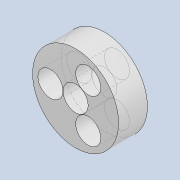
# Autodesk Inventor part: 原動節-ヘッケン接続部v2
Saved by Autodesk Inventor 2020 (Build 240168000, 168)
## iProperties
Created: 2020-06-16
Part Number: 原動節-ヘッケン接続部v2
Material: アルミニウム 2014-T4
Document SubType Name: Modeling
Designer: happy
Density: 2.8 g/cm^3
Appearance: サテン
Mass: 0.939484 g
Surface Area: 4.6873 cm^2
Volume: 0.33553 cm^3
Author: happy
Autodesk Inventor part; units mm, degrees
ref_plane "YZ Plane" through (0, 0, 0) normal (1, 0, 0) x (0, 1, 0)
ref_plane "XZ Plane" through (0, 0, 0) normal (0, 1, 0) x (-1, 0, 0)
ref_plane "XY Plane" through (0, 0, 0) normal (0, 0, 1) x (1, 0, 0)
sketch "スケッチ1" plane through (0, 0, 0) normal (0, 0, 1) x (1, 0, 0)
  circle A0 centre (0, 0) radius 1.74
  circle A1 centre (1.75, 3.0311) radius 1.74
  circle A2 centre (-3.5, 0) radius 1.74
  circle A3 centre (1.75, -3.0311) radius 1.74
  circle A4 centre (0, 0) radius 5.975
  circle A5 centre (0, 0) radius 1.25 construction
  line L0 (-3.5, 0) -> (1.75, 3.0311) construction
  line L1 (1.75, 3.0311) -> (1.75, -3.0311) construction
  line L2 (1.75, -3.0311) -> (-3.5, 0) construction
  line L3 (0, 0) -> (3.1471, 0) construction
  circle A6 centre (0, 0) radius 3.5 construction
  dimension "d0" = 11.95
  dimension "d1" = 3.48
  dimension "d2" = 3.48
  dimension "d3" = 3.5
  constraints: 8 end point, 7 centre point, 3 point on circle, 2 coincident, 2 equal length, 2 equal radius, 1 concentric, 1 horizontal, 1 point on line, 2 other
  measures "d0" diameter of A4
  measures "d1" diameter of A0
  measures "d2" diameter of A1
  measures "d3" distance of point (0, 0) L0.start
extrude "押し出し1" add sketch "スケッチ1" along normal blind 4
equation "\"d1\" = d2"
equation "\"d3\" = d5"
equation "\"d5\" = d6"
equation "\"d6\" = 3.5"
